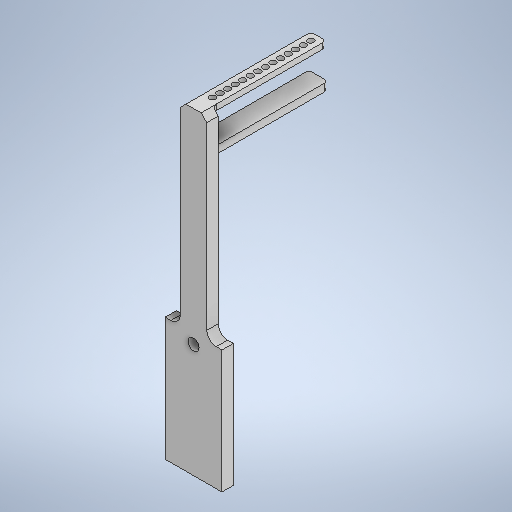
# Autodesk Inventor part: leds_holder
Saved by Autodesk Inventor 2025.2 (Build 292293000, 293)
## iProperties
Created: 2025-11-25
Part Number: leds_holder
Material: Generic
Document SubType Name: Modeling
Designer: die02
Density: 1 g/cm^3
Appearance: Default
Author: die02
Autodesk Inventor part; units mm, degrees
ref_plane "YZ Plane" through (0, 0, 0) normal (1, 0, 0) x (0, 1, 0)
ref_plane "XZ Plane" through (0, 0, 0) normal (0, 1, 0) x (-1, 0, 0)
ref_plane "XY Plane" through (0, 0, 0) normal (0, 0, 1) x (1, 0, 0)
sketch "Sketch1" plane through (0, 0, 0) normal (0, 1, 0) x (-1, 0, 0)
  line L0 (-4, 30) -> (4, 30)
  line L1 (4, 30) -> (4, -30)
  line L2 (4, -30) -> (-4, -30)
  line L3 (-4, -30) -> (-4, 30)
  line L4 (-4, 30) -> (4, -30) construction
  line L5 (4, 30) -> (-4, -30) construction
  circle A0 centre (0, 14) radius 1.6
  circle A1 centre (0, 10) radius 1.6
  circle A2 centre (0, 6) radius 1.6
  circle A3 centre (0, 2) radius 1.6
  circle A4 centre (0, -2) radius 1.6
  circle A5 centre (0, -6) radius 1.6
  circle A6 centre (0, -14) radius 1.6
  circle A7 centre (0, -10) radius 1.6
  circle A8 centre (0, 26) radius 1.6
  circle A9 centre (0, 22) radius 1.6
  circle A10 centre (0, 18) radius 1.6
  circle A11 centre (0, -18) radius 1.6
  circle A12 centre (0, -26) radius 1.6
  circle A13 centre (0, -22) radius 1.6
  point P0 (0, 0)
  dimension "d0" = 3.2
  dimension "d1" = 3.2
  dimension "d2" = 3.2
  dimension "d3" = 3.2
  dimension "d5" = 3.2
  dimension "d6" = 3.2
  dimension "d7" = 3.2
  dimension "d8" = 3.2
  dimension "d9" = 3.2
  dimension "d10" = 3.2
  dimension "d11" = 3.2
  dimension "d12" = 3.2
  dimension "d13" = 3.2
  dimension "d14" = 3.2
  dimension "d15" = 4
  dimension "d16" = 4
  dimension "d17" = 4
  dimension "d18" = 4
  dimension "d19" = 4
  dimension "d20" = 4
  dimension "d21" = 4
  dimension "d22" = 4
  dimension "d23" = 4
  dimension "d24" = 4
  dimension "d25" = 4
  dimension "d26" = 4
  dimension "d27" = 4
  dimension "d28" = 4
  dimension "d29" = 4
  dimension "d30" = 4
  dimension "d31" = 4
  dimension "d32" = 30
  constraints: 14 centre point, 12 end point, 2 midpoint, 2 parallel, 1 horizontal, 1 perpendicular
  measures "d0" diameter of A0
  measures "d1" diameter of A1
  measures "d2" diameter of A2
  measures "d3" diameter of A3
  measures "d5" diameter of A4
  measures "d6" diameter of A5
  measures "d7" diameter of A6
  measures "d8" diameter of A7
  measures "d9" diameter of A8
  measures "d10" diameter of A9
  measures "d11" diameter of A10
  measures "d12" diameter of A11
  measures "d13" diameter of A12
  measures "d14" diameter of A13
  measures "d15" distance of A9.centre A8.centre
  measures "d16" distance of A10.centre A9.centre
  measures "d17" distance of A10.centre A0.centre
  measures "d18" distance of A1.centre A0.centre
  measures "d19" distance of A2.centre A1.centre
  measures "d20" distance of A3.centre A2.centre
  measures "d21" distance of A3.centre A4.centre
  measures "d22" distance of A4.centre A5.centre
  measures "d23" distance of A5.centre A7.centre
  measures "d24" distance of A7.centre A6.centre
  measures "d25" distance of A6.centre A11.centre
  measures "d26" distance of A11.centre A13.centre
  measures "d27" distance of A12.centre A13.centre
  measures "d28" distance from line of A8.centre L0
  measures "d29" distance from line of L2 A12.centre
  measures "d30" distance from line of A12.centre L1
  measures "d31" distance from line of A12.centre L3
  measures "d32" distance from line of point (0, 0) L0
extrude "Extrusion1" add sketch "Sketch1" along normal blind 3
fillet "Fillet1" radius 2 2 edges at (4, 1.5, -30) (-4, 1.5, -30)
sketch "Sketch4" plane through (-4, 0, 30) normal (0, 0, 1) x (1, 0, 0)
  line L0 (8, 0) -> (8, 3) projected
  line L1 (0, 0) -> (0, 3) projected
  line L2 (8, 0) -> (0, 0)
  line L3 (0, 0) -> (0, 3)
  line L4 (0, 3) -> (8, 3)
  line L5 (8, 3) -> (8, 0)
  point P0 (4, 0)
  constraints: 8 end point, 2 parallel, 1 horizontal, 1 perpendicular
extrude "Extrusion4" add sketch "Sketch4" along normal blind 6
sketch "Sketch5" plane through (0, 0, 0) normal (0, -1, 0) x (1, 0, 0)
  line L0 (7, 36) -> (-7, 36)
  line L1 (-7, 36) -> (-7, 30)
  line L2 (-7, 30) -> (7, 30)
  line L3 (7, 30) -> (7, 36)
  line L4 (-4, 36) -> (4, 36) projected
  line L5 (4, -28) -> (4, 36) projected
  line L6 (-4, -28) -> (-4, 36) projected
  point P0 (0, 0)
  dimension "d51" = 0
  dimension "d52" = 3
  dimension "d53" = 3
  dimension "d54" = 6
  constraints: 8 end point, 2 parallel, 1 horizontal, 1 perpendicular
  measures "d51" distance between parallel lines of L4 L0
  measures "d52" distance between parallel lines of L5 L3
  measures "d53" distance between parallel lines of L6 L1
  measures "d54" distance between parallel lines of L0 L2
extrude "Extrusion5" add sketch "Sketch5" along normal blind 100
chamfer "Chamfer1" distance 3 angle 45 2 edges at (4, 0, 33) (-4, 0, 33)
sketch "Sketch6" plane through (4, 0, 30) normal (0, 0, -1) x (-1, 0, 0)
  line L0 (9, -15) -> (-1, -15)
  line L1 (-1, -15) -> (-1, -19)
  line L2 (-1, -19) -> (9, -19)
  line L3 (9, -19) -> (9, -15)
  line L4 (-3, 0) -> (-3, -100) projected
  line L5 (11, 0) -> (11, -100) projected
  line L6 (2, 0) -> (0, 0) projected
  point P0 (4, 0)
  dimension "d60" = 2
  dimension "d61" = 2
  dimension "d62" = 15
  dimension "d63" = 4
  constraints: 8 end point, 2 parallel, 1 horizontal, 1 perpendicular
  measures "d60" distance between parallel lines of L4 L1
  measures "d61" distance between parallel lines of L5 L3
  measures "d62" distance between parallel lines of L6 L0
  measures "d63" distance between parallel lines of L0 L2
extrude "Extrusion6" add sketch "Sketch6" along normal up to surface (60 mm away)
fillet "Fillet3" radius 2 2 edges at (5, -17, -30) (-5, -17, -30)
fillet "Fillet4" radius 2 1 edges at (-4, 1.5, 30)
fillet "Fillet5" radius 2 2 edges at (4, 1.5, 30) (5, -17, 30)
fillet "Fillet6" radius 2 1 edges at (-5, -17, 30)
sketch "Sketch7" plane through (0, -100, 0) normal (0, -1, 0) x (1, 0, 0)
  line L0 (-15, 36) -> (15, 36)
  line L1 (15, 36) -> (15, 30)
  line L2 (15, 30) -> (-15, 30)
  line L3 (-15, 30) -> (-15, 36)
  line L4 (-7, 30) -> (7, 30) projected
  line L5 (-7, 36) -> (-7, 30) projected
  point P0 (0, 0)
  point P1 (-15, 33)
  point P2 (0, 30)
  dimension "d70" = 0
  dimension "d72" = 30
  dimension "d73" = 15
  dimension "d74" = 6
  constraints: 8 end point, 2 midpoint, 2 parallel, 1 horizontal, 1 perpendicular
  measures "d70" distance between parallel lines of L4 L2
  measures "d72" distance between parallel lines of L3 L1
  measures "d73" distance from line of L1 point (0, 30)
  measures "d74" distance between parallel lines of L2 L0
extrude "Extrusion7" add sketch "Sketch7" along normal blind 65
sketch "Sketch8" plane through (-4, 0, 36) normal (0, 0, 1) x (1, 0, 0)
  circle A0 centre (4, -105) radius 2.95
  line L0 (-11, -100) -> (-11, -165) projected
  line L1 (19, -165) -> (-11, -165) projected
  point P0 (4, 0)
  dimension "d77" = 5.9
  dimension "d79" = 15
  dimension "d80" = 60
  constraints: 1 centre point
  measures "d77" diameter of A0
  measures "d79" distance from line of L0 A0.centre
  measures "d80" distance from line of L1 A0.centre
extrude "Extrusion8" cut sketch "Sketch8" against normal blind 65
fillet "Fillet7" radius 5 1 edges at (-7, -100, 33)
fillet "Fillet8" radius 5 1 edges at (7, -100, 33)
body "Solid1"
